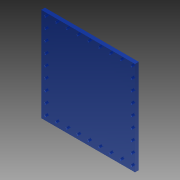
# Autodesk Inventor part: tray
Saved by Autodesk Inventor 2014 SP2 (Build 180246200, 246)
## iProperties
Created: 2016-09-18
Part Number: tray
Material: Generic
Document SubType Name: Modeling
Designer: cruiser
Density: 1 g/cm^3
Appearance: Default
Mass: 132.3 g
Surface Area: 485.28 cm^2
Volume: 132.3 cm^3
Author: cruiser
Autodesk Inventor part; units mm, degrees
ref_plane "YZ Plane" through (0, 0, 0) normal (1, 0, 0) x (0, 1, 0)
ref_plane "XZ Plane" through (0, 0, 0) normal (0, 1, 0) x (-1, 0, 0)
ref_plane "XY Plane" through (0, 0, 0) normal (0, 0, 1) x (1, 0, 0)
sketch "Sketch1" plane through (0, 0, 0) normal (0, 1, 0) x (-1, 0, 0)
  line L0 (-75, -75) -> (75, -75)
  line L1 (75, -75) -> (75, 75)
  line L2 (75, 75) -> (-75, 75)
  line L3 (-75, 75) -> (-75, -75)
  line L4 (-75, -75) -> (75, 75) construction
  line L5 (75, -75) -> (-75, 75) construction
  point P0 (0, 0)
  dimension "d0" = 150
  dimension "d1" = 150
  constraints: 12 end point, 2 midpoint, 2 parallel, 1 horizontal, 1 perpendicular
  measures "d0" distance of L2.end L1.end
  measures "d1" distance of L1.end L0.end
extrude "Extrusion1" add sketch "Sketch1" along normal blind 5.88
sketch "Sketch2" plane through (0, 0, 0) normal (0, -1, 0) x (1, 0, 0)
  line L0 (75, -75) -> (-75, -75) projected
  line L1 (75, 75) -> (75, -75) projected
  line L2 (-75, 75) -> (75, 75) projected
  line L3 (-75, -75) -> (-75, 75) projected
  line L4 (-73.4125, -73.4125) -> (73.4125, -73.4125)
  line L5 (73.4125, -73.4125) -> (73.4125, 73.4125)
  line L6 (73.4125, 73.4125) -> (-73.4125, 73.4125)
  line L7 (-73.4125, 73.4125) -> (-73.4125, -73.4125)
  line L8 (-73.4125, -73.4125) -> (73.4125, 73.4125) construction
  line L9 (73.4125, -73.4125) -> (-73.4125, 73.4125) construction
  line L10 (-60, -60) -> (60, -60)
  line L11 (60, -60) -> (60, 60)
  line L12 (60, 60) -> (-60, 60)
  line L13 (-60, 60) -> (-60, -60)
  line L14 (-60, -60) -> (60, 60) construction
  line L15 (60, -60) -> (-60, 60) construction
  circle A0 centre (-67.5, 67.5) radius 1.5
  circle A1 centre (-50.625, 67.5) radius 1.5
  circle A2 centre (-33.75, 67.5) radius 1.5
  circle A3 centre (-16.875, 67.5) radius 1.5
  circle A4 centre (0, 67.5) radius 1.5
  circle A5 centre (16.875, 67.5) radius 1.5
  circle A6 centre (33.75, 67.5) radius 1.5
  circle A7 centre (50.625, 67.5) radius 1.5
  circle A8 centre (67.5, 67.5) radius 1.5
  circle A9 centre (-67.5, 50.625) radius 1.5
  circle A10 centre (-50.625, 50.625) radius 1.5
  circle A11 centre (-33.75, 50.625) radius 1.5
  circle A12 centre (-16.875, 50.625) radius 1.5
  circle A13 centre (0, 50.625) radius 1.5
  circle A14 centre (16.875, 50.625) radius 1.5
  circle A15 centre (33.75, 50.625) radius 1.5
  circle A16 centre (50.625, 50.625) radius 1.5
  circle A17 centre (67.5, 50.625) radius 1.5
  circle A18 centre (-67.5, 33.75) radius 1.5
  circle A19 centre (-50.625, 33.75) radius 1.5
  circle A20 centre (-33.75, 33.75) radius 1.5
  circle A21 centre (-16.875, 33.75) radius 1.5
  circle A22 centre (0, 33.75) radius 1.5
  circle A23 centre (16.875, 33.75) radius 1.5
  circle A24 centre (33.75, 33.75) radius 1.5
  circle A25 centre (50.625, 33.75) radius 1.5
  circle A26 centre (67.5, 33.75) radius 1.5
  circle A27 centre (-67.5, 16.875) radius 1.5
  circle A28 centre (-50.625, 16.875) radius 1.5
  circle A29 centre (-33.75, 16.875) radius 1.5
  circle A30 centre (-16.875, 16.875) radius 1.5
  circle A31 centre (0, 16.875) radius 1.5
  circle A32 centre (16.875, 16.875) radius 1.5
  circle A33 centre (33.75, 16.875) radius 1.5
  circle A34 centre (50.625, 16.875) radius 1.5
  circle A35 centre (67.5, 16.875) radius 1.5
  circle A36 centre (-67.5, 0) radius 1.5
  circle A37 centre (-50.625, 0) radius 1.5
  circle A38 centre (-33.75, 0) radius 1.5
  circle A39 centre (-16.875, 0) radius 1.5
  circle A40 centre (0, 0) radius 1.5
  circle A41 centre (16.875, 0) radius 1.5
  circle A42 centre (33.75, 0) radius 1.5
  circle A43 centre (50.625, 0) radius 1.5
  circle A44 centre (67.5, 0) radius 1.5
  circle A45 centre (-67.5, -16.875) radius 1.5
  circle A46 centre (-50.625, -16.875) radius 1.5
  circle A47 centre (-33.75, -16.875) radius 1.5
  circle A48 centre (-16.875, -16.875) radius 1.5
  circle A49 centre (0, -16.875) radius 1.5
  circle A50 centre (16.875, -16.875) radius 1.5
  circle A51 centre (33.75, -16.875) radius 1.5
  circle A52 centre (50.625, -16.875) radius 1.5
  circle A53 centre (67.5, -16.875) radius 1.5
  circle A54 centre (-67.5, -33.75) radius 1.5
  circle A55 centre (-50.625, -33.75) radius 1.5
  circle A56 centre (-33.75, -33.75) radius 1.5
  circle A57 centre (-16.875, -33.75) radius 1.5
  circle A58 centre (0, -33.75) radius 1.5
  circle A59 centre (16.875, -33.75) radius 1.5
  circle A60 centre (33.75, -33.75) radius 1.5
  circle A61 centre (50.625, -33.75) radius 1.5
  circle A62 centre (67.5, -33.75) radius 1.5
  circle A63 centre (-67.5, -50.625) radius 1.5
  circle A64 centre (-50.625, -50.625) radius 1.5
  circle A65 centre (-33.75, -50.625) radius 1.5
  circle A66 centre (-16.875, -50.625) radius 1.5
  circle A67 centre (0, -50.625) radius 1.5
  circle A68 centre (16.875, -50.625) radius 1.5
  circle A69 centre (33.75, -50.625) radius 1.5
  circle A70 centre (50.625, -50.625) radius 1.5
  circle A71 centre (67.5, -50.625) radius 1.5
  circle A72 centre (-67.5, -67.5) radius 1.5
  circle A73 centre (-50.625, -67.5) radius 1.5
  circle A74 centre (-33.75, -67.5) radius 1.5
  circle A75 centre (-16.875, -67.5) radius 1.5
  circle A76 centre (0, -67.5) radius 1.5
  circle A77 centre (16.875, -67.5) radius 1.5
  circle A78 centre (33.75, -67.5) radius 1.5
  circle A79 centre (50.625, -67.5) radius 1.5
  circle A80 centre (67.5, -67.5) radius 1.5
  point P0 (0, 0)
  dimension "d4" = 146.825
  dimension "d5" = 146.825
  dimension "d6" = 120
  dimension "d7" = 120
  dimension "d8" = 3
  dimension "d9" = 7.5
  dimension "d10" = 7.5
  dimension "d13" = 16.875
  dimension "d16" = 16.875
  constraints: 81 centre point, 24 end point, 4 midpoint, 4 parallel, 3 horizontal, 2 perpendicular, 1 vertical, 160 other
  measures "d4" distance of L6.end L5.end
  measures "d5" distance of L6.end L4.start
  measures "d6" distance of L12.end L11.end
  measures "d7" distance of L11.end L10.end
  measures "d8" diameter of A0
  measures "d9" distance from line of L12 A0.centre
  measures "d10" distance from line of L13 A0.centre
  measures "d13" distance of A0.centre A1.centre
  measures "d16" distance of A0.centre A9.centre
extrude "Extrusion2" cut sketch "Sketch2" against normal up to next contours L0 L3 L2 L1 | A0 | A1 | A2 | A3 | A4 | A5 | A6 | A7 | A8 | A9 | A17 | A18 | A26 | A27 | A35 | A36 | A44 | A45 | A53 | A54 | A62 | A63 | A71 | A72 | A73 | A74 | A75 | A76 | A77 | A78 | A79 | A80
equation "\"d0\" = tray_x"
equation "\"d1\" = tray_y"
equation "\"d2\" = tray_t"
equation "\"d4\" = tray_x - 4 * reservoir_t"
equation "\"d5\" = tray_y - 4 * reservoir_t"
equation "\"d6\" = reservoir_opening_x"
equation "\"d7\" = reservoir_opening_y"
equation "\"d8\" = m3_diameter"
equation "\"d9\" = -0.25 * reservoir_opening_y + 0.25 * reservoir_y"
equation "\"d10\" = -0.25 * reservoir_opening_x + 0.25 * reservoir_x"
equation "\"d13\" = 0.0625 * reservoir_opening_x + 0.0625 * reservoir_x"
equation "\"d16\" = 0.0625 * reservoir_opening_y + 0.0625 * reservoir_y"
equation "\"laserresin\" = 5"
equation "\"st1_thickness\" = 0.91186"
equation "\"st2_thickness\" = 1.5875"
equation "\"st3_thickness\" = 1.5875"
equation "\"al1_thickness\" = 0.79375"
equation "\"al2_thickness\" = 1.5875"
equation "\"al3_thickness\" = 1.5875"
equation "\"bend_factor\" = 2.26205"
equation "\"st1_bend\" = 2.06267"
equation "\"st2_bend\" = 3.591"
equation "\"st3_bend\" = 3.591"
equation "\"al1_bend\" = 1.7955"
equation "\"al2_bend\" = 3.591"
equation "\"al3_bend\" = 3.591"
equation "\"acrylic1_thickness\" = 5.88"
equation "\"acrylic2_thickness\" = 3.15"
equation "\"acrylic3_thickness\" = 3.15"
equation "\"nema17_x\" = 43"
equation "\"switch_spacing\" = 19"
equation "\"laser_body_diameter\" = 12"
equation "\"m3_diameter\" = 3"
equation "\"m3_head\" = 6"
equation "\"m4_diameter\" = 4"
equation "\"m5_diameter\" = 5"
equation "\"m5_head\" = 10.3"
equation "\"rivet_diameter\" = 3.3"
equation "\"brass_insert_drill\" = 4"
equation "\"m5_brass_insert_drill\" = 6.7"
equation "\"m3_press_nut_drill\" = 4.5"
equation "\"m5_press_nut_drill\" = 6.5"
equation "\"linear_bearing_spacing\" = 209"
equation "\"platform_t\" = 1.5875"
equation "\"platform_z\" = 65"
equation "\"platform_fold_x\" = 15"
equation "\"platform_crane_gap\" = 0.1"
equation "\"platform_upper_y\" = 46.625"
equation "\"crane_t\" = 1.5875"
equation "\"crane_x\" = 234"
equation "\"crane_gap\" = 0.1"
equation "\"tray_t\" = 5.88"
equation "\"tray_x\" = 150"
equation "\"tray_y\" = 150"
equation "\"reservoir_t\" = 0.79375"
equation "\"reservoir_z\" = 35"
equation "\"frame_front_t\" = 0.91186"
equation "\"frame_front_x\" = 280.23622"
equation "\"frame_front_y\" = 56"
equation "\"frame_gap\" = 0.1"
equation "\"frame_back_t\" = 0.91186"
equation "\"frame_back_x\" = 278.2125"
equation "\"frame_back_y\" = 53.97628"
equation "\"frame_back_z\" = 497.97628"
equation "\"frame_opening_x\" = 200.23622"
equation "\"drawer_t\" = 0.79375"
equation "\"drawer_x\" = 202.02372"
equation "\"drawer_y\" = 73"
equation "\"dawer_top_y\" = 0"
equation "\"foot_t\" = 1.5875"
equation "\"foot_x\" = 199"
equation "\"foot_y\" = 196"
equation "\"reservoir_opening_y\" = 120"
equation "\"reservoir_opening_x\" = 120"
equation "\"nema17_shaft\" = 24"
equation "\"drawer_window_gap\" = 6"
equation "\"reservoir_flap_y\" = 20.79375"
equation "\"drawer_seal_y\" = 101"
equation "\"drawer_gap\" = 0.1"
equation "\"tray_to_platform_oversize\" = 0"
equation "\"lmk8uu_shaft\" = 15"
equation "\"lmk8uu_x\" = 25"
equation "\"lmk8uu_z\" = 24"
equation "\"drawer_reservoir_overlap_x\" = 24.20625"
equation "\"frame_front_fold\" = 15"
equation "\"shf8_y\" = 43"
equation "\"acme_nut_d\" = 19.1"
equation "\"acme_nut_upper_d\" = 12.7"
equation "\"handle_spacing\" = 50.8"
equation "\"handle_projection\" = 20.6375"
equation "\"handle_hole_d\" = 5.0625"
equation "\"handle_d\" = 4.7625"
equation "\"laser_offset_x\" = 59.5"
equation "\"laser_holder_z\" = 75"
equation "\"laser_holder_t\" = 0.79375"
equation "\"subframe_y\" = 55"
equation "\"subframe_t\" = 0.79375"
equation "\"subframe_x\" = 66"
equation "\"laser_offset_y\" = 8.5"
equation "\"galvo_y_in_offset\" = 17.5"
equation "\"galvo_y_out_offset\" = 27"
equation "\"laser_diameter\" = 13"
equation "\"corner_big_r\" = 5"
equation "\"corner_small_r\" = 1"
equation "\"rivet2_diameter\" = 3.26"
equation "\"rivet1_diameter\" = 3.26"
equation "\"platform_gap\" = 0.1"
equation "\"shield_z\" = 260.79375"
equation "\"shield_x\" = 200.43622"
equation "\"shield_y\" = 71"
equation "\"shield_t\" = 3.15"
equation "\"magnet_t\" = 2"
equation "\"reservoir_y\" = 150"
equation "\"reservoir_x\" = 150"
body "Solid1"
